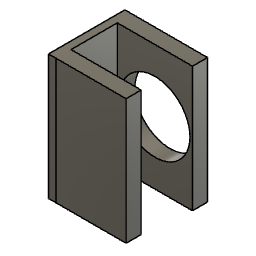
AmbientLightHolder v1 (Autodesk Fusion 360 design; units mm, degrees)
Autodesk Fusion 360 part; units mm, degrees
sketch "Sketch1" plane through (0, 0, 0) normal (0, 1, 0) x (1, 0, 0)
  line L0 (-7.5, 7.625) -> (7.5, 7.625)
  line L1 (7.5, 7.625) -> (7.5, 4.625)
  line L2 (7.5, 4.625) -> (-7.5, 4.625)
  line L3 (-7.5, 4.625) -> (-7.5, 7.625)
  line L4 (-7.5, -4.625) -> (6.5, -4.625)
  line L5 (6.5, -4.625) -> (6.5, -7.625)
  line L6 (6.5, -7.625) -> (-7.5, -7.625)
  line L7 (-7.5, -7.625) -> (-7.5, -4.625)
  line L8 (-7.5, 7.625) -> (-9, 7.625)
  line L9 (-9, 7.625) -> (-9, -7.6278)
  line L10 (-9, -7.6278) -> (-7.5, -7.6278)
  line L11 (-7.5, -7.6278) -> (-7.5, 7.625)
  dimension "d3" = 4.625
  dimension "d4" = 4.625
  dimension "d5" = 15
  dimension "d6" = 7.5
  dimension "d7" = 14
  dimension "d9" = 7.5
  dimension "d10" = 1.5
  constraint horizontal L0
  constraint vertical L1
  constraint horizontal L2
  constraint vertical L3
  constraint horizontal L4
  constraint vertical L5
  constraint horizontal L6
  constraint vertical L7
  constraint horizontal L8
  constraint vertical L9
  constraint horizontal L10
  constraint vertical L11
  measures "d3" vertical distance of origin L2.end
  measures "d4" vertical distance of origin L4.start
  measures "d5" distance of L0.start L0.end
  measures "d6" horizontal distance of origin L2.end
  measures "d7" distance of L5.end L6.end
  measures "d9" horizontal distance of origin L4.start
  measures "d10" distance of L0.start L8.end
extrude "Extrude1" add sketch "Sketch1" along normal blind 25
sketch "Sketch2" plane through (0, 0, -7.625) normal (0, 0, -1) x (-1, 0, 0)
  line L0 (-7.5, 0) -> (9, 0)
  line L1 (9, 0) -> (9, 25)
  line L2 (9, 25) -> (-7.5, 25)
  line L3 (-7.5, 25) -> (-7.5, 0)
  circle A0 centre (0, 12.5) radius 7
  dimension "d13" = 9
  dimension "d14" = 14
  dimension "d15" = 12.5
  measures "d13" horizontal distance of L0.end A0.centre
  measures "d14" diameter of A0
  measures "d15" vertical distance of L0.end A0.centre
extrude "Extrude2" cut sketch "Sketch2" against normal blind 9 contours A0
equation "d3 = ( 9.25 / 2 ) * 1 mm"
equation "d4 = ( 9.25 / 2 ) * 1 mm"
